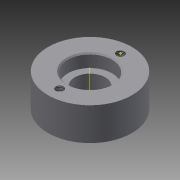
# Autodesk Inventor part: Корпус
Saved by Autodesk Inventor 2015 SP1 (Build 190203100, 203)
## iProperties
Created: 2019-05-12
Part Number: Корпус
Material: Типовые
Document SubType Name: Modeling
Density: 1 g/cm^3
Appearance: По умолчанию
Mass: 303.652 g
Surface Area: 406.671 cm^2
Volume: 303.652 cm^3
Autodesk Inventor part; units mm, degrees
ref_plane "YZ Plane" through (0, 0, 0) normal (1, 0, 0) x (0, 1, 0)
ref_plane "XZ Plane" through (0, 0, 0) normal (0, 1, 0) x (-1, 0, 0)
ref_plane "XY Plane" through (0, 0, 0) normal (0, 0, 1) x (1, 0, 0)
sketch "Эскиз1" plane through (0, 0, 0) normal (0, 0, 1) x (1, 0, 0)
  circle A0 centre (0, 0) radius 55
  circle A1 centre (0, 0) radius 20
  dimension "d0" = 110
  dimension "d1" = 40
  constraints: 2 centre point, 2 coincident
  measures "d0" diameter of A0
  measures "d1" diameter of A1
extrude "Выдавливание1" add sketch "Эскиз1" along normal blind 43
sketch "Эскиз2" plane through (0, 0, 43) normal (0, 0, 1) x (1, 0, 0)
  circle A0 centre (0, 0) radius 55 projected
  circle A1 centre (0, 0) radius 29
  dimension "d6" = 58
  constraints: 1 centre point, 1 coincident
  measures "d6" diameter of A1
extrude "Выдавливание2" cut sketch "Эскиз2" against normal blind 17 contours A1
sketch "Эскиз3" plane through (0, 0, 0) normal (0, 0, -1) x (-1, 0, 0)
  circle A0 centre (0, 0) radius 31
  dimension "d9" = 62
  constraints: 1 centre point, 1 coincident
  measures "d9" diameter of A0
extrude "Выдавливание3" cut sketch "Эскиз3" against normal blind 11
sketch "Эскиз4" plane through (0, 0, 43) normal (0, 0, 1) x (1, 0, 0)
  circle A0 centre (0, 0) radius 40
  line L0 (0, 0) -> (0, 40)
  circle A1 centre (0, 0) radius 55 projected
  dimension "d12" = 80
  constraints: 2 end point, 1 coincident, 1 vertical, 1 vertical alignment, 2 other
hole "Отверстие1" at (0, 40, 43) direction (0, 0, -1) diameter 10.106 depth 38.3 tip angle 118 thread size "M12x1.75" class "6H" standard "ANSI Metric M Profile"
pattern_circular "Круговой массив1" count 2 over 360 about axis through (0, 0, 11) along (0, 0, -1) of "Отверстие1"
chamfer "Фаска2" distance 1.6 angle 45 1 edges at (-29, 0, 43)
sketch "Эскиз5" plane through (0, 0, 43) normal (0, 0, 1) x (1, 0, 0)
  point P0 (0, 40)
  point P1 (-62.4077, 41.077)
